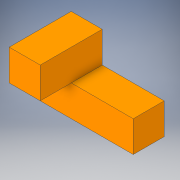
# Autodesk Inventor part: Orange part
Saved by Autodesk Inventor 2017 (Build 210142000, 142)
## iProperties
Created: 2016-11-02
Part Number: Orange part
Material: Generic
Document SubType Name: Modeling
Designer: rbibb
Density: 1 g/cm^3
Appearance: Default
Author: rbibb
Autodesk Inventor part; units mm, degrees
ref_plane "YZ Plane" through (0, 0, 0) normal (1, 0, 0) x (0, 1, 0)
ref_plane "XZ Plane" through (0, 0, 0) normal (0, 1, 0) x (-1, 0, 0)
ref_plane "XY Plane" through (0, 0, 0) normal (0, 0, 1) x (1, 0, 0)
sketch "Sketch1" plane through (0, 0, 0) normal (1, 0, 0) x (0, 1, 0)
  point P0 (0, 0)
sketch "Sketch2" plane through (0, 0, 0) normal (1, 0, 0) x (0, 1, 0)
  point P0 (0, 0)
sketch "Sketch3" plane through (0, 0, 0) normal (1, 0, 0) x (0, 1, 0)
  line L0 (12.8972, 23.077) -> (-6.1528, 23.077)
  line L1 (-6.1528, 23.077) -> (-6.1528, 4.027)
  line L2 (-6.1528, 4.027) -> (12.8972, 4.027)
  line L3 (12.8972, 4.027) -> (12.8972, 23.077)
  point P0 (0, 0)
  dimension "d0" = 19.05
  dimension "d1" = 19.05
  constraints: 8 end point, 2 parallel, 1 horizontal, 1 perpendicular
  measures "d0" distance of L2.end L1.end
  measures "d1" distance of L1.end L0.end
extrude "Extrusion1" add sketch "Sketch3" along normal blind 57.15
sketch "Sketch4" plane through (0, 12.8972, 23.077) normal (0, 1, 0) x (1, 0, 0)
  line L0 (0, 0) -> (0, 19.05) projected
  line L1 (0, 19.05) -> (57.15, 19.05) projected
  line L2 (0, 0) -> (19.05, 0)
  line L3 (19.05, 0) -> (19.05, 19.05)
  line L4 (19.05, 19.05) -> (0, 19.05)
  line L5 (0, 19.05) -> (0, 0)
  point P0 (0, 23.077)
  dimension "d4" = 19.05
  constraints: 8 end point, 2 parallel, 1 horizontal, 1 perpendicular, 1 point on line
  measures "d4" distance of L4.end L3.end
extrude "Extrusion2" add sketch "Sketch4" along normal blind 19.05
sketch "Sketch5" plane through (0, -6.1528, 23.077) normal (0, 0, 1) x (1, 0, 0)
  line L0 (19.05, 38.1) -> (0, 38.1) projected
  line L1 (19.05, 19.05) -> (19.05, 38.1) projected
  line L2 (0, 38.1) -> (19.05, 38.1)
  line L3 (19.05, 38.1) -> (19.05, 19.05)
  line L4 (19.05, 19.05) -> (0, 19.05)
  line L5 (0, 19.05) -> (0, 38.1)
  point P0 (0, 6.1528)
  constraints: 8 end point, 2 parallel, 1 horizontal, 1 perpendicular
extrude "Extrusion3" add sketch "Sketch5" along normal blind 19.05
body "Solid1"
